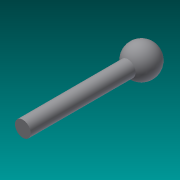
# Autodesk Inventor part: pin kepala
Saved by Autodesk Inventor 2014 SP2 (Build 180246200, 246)
## iProperties
Created: 2019-08-02
Part Number: pin kepala
Material: Generic
Document SubType Name: Modeling
Designer: USER PC
Density: 1 g/cm^3
Appearance: Default
Author: USER PC
Autodesk Inventor part; units mm, degrees
ref_plane "YZ Plane" through (0, 0, 0) normal (1, 0, 0) x (0, 1, 0)
ref_plane "XZ Plane" through (0, 0, 0) normal (0, 1, 0) x (-1, 0, 0)
ref_plane "XY Plane" through (0, 0, 0) normal (0, 0, 1) x (1, 0, 0)
sketch "Sketch1" plane through (0, 0, 0) normal (0, 0, 1) x (1, 0, 0)
  line L0 (0, 0) -> (15, 0)
  line L1 (15, 0) -> (15, -200)
  line L2 (15, -200) -> (0, -200)
  line L3 (0, -200) -> (0, 0)
  dimension "d0" = 15
  dimension "d1" = 200
  constraints: 8 end point, 2 parallel, 1 horizontal, 1 perpendicular
  measures "d0" distance of L1.end L2.end
  measures "d1" distance of L0.end L1.end
revolve "Revolution1" add sketch "Sketch1" angle 360 about axis through (0, -200, 0) along (0, 1, 0)
sketch "Sketch2" plane through (0, 0, 0) normal (0, 0, 1) x (1, 0, 0)
  arc A0 (0, -4.1079) -> (0, 55.8921) centre (0, 25.8921) ccw
  line L0 (0, 55.8921) -> (0, -4.1079)
  point P0 (0, 0)
  dimension "d3" = 60
  constraints: 2 end point, 2 point on circle, 1 centre point, 1 vertical
  measures "d3" diameter of A0
revolve "Revolution2" add sketch "Sketch2" angle 360 about axis through (0, 55.8921, 0) along (0, -1, 0)
body "Solid1"
